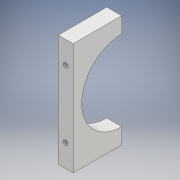
# Autodesk Inventor part: 모터받침대
Saved by Autodesk Inventor 2017 (Build 210142000, 142)
## iProperties
Part Number: 모터받침대
Material: ABS 플라스틱
Document SubType Name: Modeling
Designer: minom
Mass: 5.96395 g
Surface Area: 30.8125 cm^2
Volume: 5.62637 cm^3
Density: 1.06 g/cm^3
Appearance: 매끄러움 - 흰색
Author: minom
Autodesk Inventor part; units mm, degrees
ref_plane "YZ Plane" through (0, 0, 0) normal (1, 0, 0) x (0, 1, 0)
ref_plane "XZ Plane" through (0, 0, 0) normal (0, 1, 0) x (-1, 0, 0)
ref_plane "XY Plane" through (0, 0, 0) normal (0, 0, 1) x (1, 0, 0)
sketch "스케치1" plane through (0, 0, 0) normal (1, 0, 0) x (0, 1, 0)
  line L0 (0, 0) -> (27, 0)
  line L1 (27, -60) -> (0, -60)
  line L2 (0, -60) -> (0, 0)
  arc A0 (27, -8.5) -> (27, -51.5) centre (27, -30) ccw
  line L3 (27, 0) -> (27, -8.5)
  line L4 (27, -51.5) -> (27, -60)
  dimension "d0" = 27
  dimension "d3" = 60
  dimension "d4" = 27
  dimension "d5" = 21.5
  dimension "d6" = 27
  dimension "d7" = 30
  constraints: 10 end point, 3 parallel, 2 perpendicular, 2 point on circle, 1 centre point, 1 horizontal
  measures "d0" distance of L1.start L1.end
  measures "d3" distance between parallel lines of L1 L0
  measures "d4" distance between parallel lines of L2 L3
  measures "d5" radius of A0
  measures "d6" distance from line of L2 A0.centre
  measures "d7" distance from line of L0 A0.centre
extrude "돌출1" add sketch "스케치1" along normal blind 8
sketch "스케치2" plane through (0, 0, -60) normal (0, -1, 0) x (1, 0, 0)
  line L0 (0, 0) -> (0, 60) projected
  line L1 (0, 0) -> (8, 0) projected
  line L2 (8, 60) -> (8, 0) projected
  line L3 (0, 60) -> (8, 60) projected
  line L4 (0, 60) -> (0, 51.5) projected
  line L5 (0, 60) -> (8, 60) projected
  line L6 (8, 51.5) -> (8, 60) projected
  line L7 (0, 51.5) -> (8, 51.5) projected
  line L8 (0, 8.5) -> (0, 0) projected
  line L9 (0, 8.5) -> (8, 8.5) projected
  line L10 (8, 0) -> (8, 8.5) projected
  line L11 (0, 0) -> (8, 0) projected
  circle A0 centre (4, 48) radius 1.25
  circle A1 centre (4, 12) radius 1.25
  dimension "d10" = 2.5
  dimension "d11" = 2.5
  dimension "d12" = 4
  dimension "d13" = 4
  dimension "d14" = 12
  dimension "d15" = 12
  constraints: 2 centre point
  measures "d10" diameter of A0
  measures "d11" diameter of A1
  measures "d12" distance from line of L0 A0.centre
  measures "d13" distance from line of L2 A1.centre
  measures "d14" distance from line of A0.centre L3
  measures "d15" distance from line of L1 A1.centre
extrude "돌출2" cut sketch "스케치2" against normal blind 9 contours A0 | A1
sketch "스케치3" plane through (0, 0, -60) normal (0, -1, 0) x (1, 0, 0)
  circle A0 centre (4, 48) radius 1.25 projected
  circle A1 centre (4, 12) radius 1.25 projected
  line L0 (0, 0) -> (0, 60) projected
  line L1 (0, 0) -> (8, 0) projected
  line L2 (8, 60) -> (8, 0) projected
  line L3 (0, 60) -> (8, 60) projected
extrude "돌출3" cut sketch "스케치3" against normal blind 1
